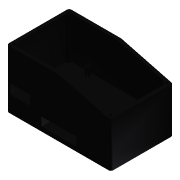
# Autodesk Inventor part: CustomBox_base
Saved by Autodesk Inventor 2013 (Build 170138000, 138)
## iProperties
Created: 2013-03-21
Part Number: CustomBox_base
Material: Generic
Document SubType Name: Modeling
Designer: Alexander
Density: 1 g/cm^3
Author: Alexander
Autodesk Inventor part; units mm, degrees
ref_plane "YZ Plane" through (0, 0, 0) normal (1, 0, 0) x (0, 1, 0)
ref_plane "XZ Plane" through (0, 0, 0) normal (0, 1, 0) x (-1, 0, 0)
sketch "Sketch1" plane through (0, 0, 0) normal (0, 1, 0) x (-1, 0, 0)
  line L0 (0, 0) -> (76.2, 0)
  line L1 (76.2, 0) -> (76.2, 45.72)
  line L2 (76.2, 45.72) -> (0, 45.72)
  line L3 (0, 45.72) -> (0, 0)
  dimension "d9" = 45.72
  dimension "d11" = 76.2
  constraints: 8 end point, 2 parallel, 1 horizontal, 1 perpendicular
  measures "d9" distance of L0.end L1.end
  measures "d11" distance of L1.end L2.end
extrude "Extrusion1" add sketch "Sketch1" along normal blind 2.54
sketch "Sketch5" plane through (0, 2.54, 0) normal (0, 1, 0) x (1, 0, 0)
  circle A0 centre (-57.15, -5.461) radius 1.5875
  circle A1 centre (-57.15, -40.259) radius 1.5875
  circle A2 centre (-6.35, -40.259) radius 1.5875
  circle A3 centre (-6.35, -5.461) radius 1.5875
  line L0 (0, 0) -> (-76.2, 0) projected
  line L1 (-76.2, 0) -> (-76.2, -45.72) projected
  line L2 (0, -45.72) -> (0, 0) projected
  line L3 (-76.2, -22.86) -> (0, -22.86)
  dimension "d8" = 3.175
  dimension "d12" = 3.175
  dimension "d13" = 3.175
  dimension "d14" = 3.175
  dimension "d15" = 34.798
  dimension "d16" = 50.8
  dimension "d32" = 5.461
  dimension "d34" = 6.35
  constraints: 4 centre point, 2 end point, 2 horizontal alignment, 2 midpoint, 2 vertical alignment
  measures "d8" diameter of A0
  measures "d12" diameter of A1
  measures "d13" diameter of A2
  measures "d14" diameter of A3
  measures "d15" distance of A1.centre A0.centre
  measures "d16" distance of A3.centre A0.centre
  measures "d32" distance from line of L0 A0.centre
  measures "d34" distance from line of L2 A2.centre
extrude "Extrusion4" add sketch "Sketch5" along normal blind 6.096 contours A0 | A1 | A2 | A3
sketch "Sketch6" plane through (0, 2.54, 0) normal (0, 1, 0) x (1, 0, 0)
  line L0 (-56.769, -39.624) -> (-6.985, -39.624)
  line L1 (-6.985, -39.624) -> (-6.985, -6.096)
  line L2 (-6.985, -6.096) -> (-56.769, -6.096)
  line L3 (-56.769, -6.096) -> (-56.769, -39.624)
  circle A0 centre (-57.15, -5.461) radius 1.5875 projected
  circle A1 centre (-57.15, -40.259) radius 1.5875 projected
  dimension "d21" = 49.784
  dimension "d22" = 33.528
  dimension "d25" = 0.381
  dimension "d27" = 0.635
  constraints: 8 end point, 2 parallel, 1 horizontal, 1 perpendicular
  measures "d21" distance of L2.end L1.end
  measures "d22" distance of L0.end L1.end
  measures "d25" distance from line of A0.centre L3
  measures "d27" distance from line of A1.centre L0
extrude "Extrusion6" cut sketch "Sketch6" along normal blind 6.35 contours L3 A1 L0 | A1 L3 A0 L2 L1 L0 | L3 L2 A0 picked at (-56.1138, -39.5193) picked at (-56.1138, -6.2007)
sketch "Sketch7" plane through (0, 2.54, 0) normal (0, 1, 0) x (1, 0, 0)
  line L0 (0, 0) -> (-76.2, 0) projected
  line L1 (-76.2, 0) -> (-76.2, -45.72) projected
  line L2 (-76.2, -45.72) -> (0, -45.72) projected
  line L3 (0, -45.72) -> (0, 0) projected
  line L4 (-72.205, -2.54) -> (-4.1275, -2.54)
  line L5 (-2.54, -4.1275) -> (-2.54, -41.5925)
  line L6 (-4.1275, -43.18) -> (-72.205, -43.18)
  line L7 (-73.66, -40.9575) -> (-73.66, -4.7625)
  arc A0 (-72.205, -43.18) -> (-73.66, -40.9575) centre (-73.66, -42.545) ccw
  arc A1 (-2.54, -41.5925) -> (-4.1275, -43.18) centre (-2.54, -43.18) ccw
  arc A2 (-4.1275, -2.54) -> (-2.54, -4.1275) centre (-2.54, -2.54) ccw
  arc A3 (-73.66, -4.7625) -> (-72.205, -2.54) centre (-73.66, -3.175) ccw
  dimension "d28" = 2.54
  dimension "d29" = 2.54
  dimension "d30" = 2.54
  dimension "d31" = 2.54
  dimension "d44" = 3.175
  dimension "d45" = 3.175
  dimension "d46" = 3.175
  dimension "d47" = 3.175
  constraints: 8 end point, 8 point on circle, 4 centre point, 2 parallel, 1 horizontal, 1 perpendicular
  measures "d28" distance between parallel lines of L0 L4
  measures "d29" distance between parallel lines of L7 L1
  measures "d30" distance between parallel lines of L2 L6
  measures "d31" distance between parallel lines of L3 L5
  measures "d44" diameter of A0
  measures "d45" diameter of A1
  measures "d46" diameter of A2
  measures "d47" diameter of A3
sketch "Sketch8" plane through (0, 8.636, 0) normal (0, 1, 0) x (1, 0, 0)
  arc A0 (-55.695, -6.096) -> (-56.769, -7.0021) centre (-57.15, -5.461) ccw projected
  arc A1 (-56.769, -38.7179) -> (-55.695, -39.624) centre (-57.15, -40.259) ccw projected
  arc A2 (-7.805, -39.624) -> (-6.985, -38.804) centre (-6.35, -40.259) ccw projected
  arc A3 (-6.985, -6.916) -> (-7.805, -6.096) centre (-6.35, -5.461) ccw projected
  point P0 (0, 0)
  constraints: 4 coincident
hole "Hole1" at (-57.15, 8.636, 5.461) at (-57.15, 8.636, 40.259) at (-6.35, 8.636, 40.259) at (-6.35, 8.636, 5.461) direction (0, -1, 0) diameter 1.6 depth 6.35 tip angle 118
fillet "Fillet1" radius 1.5875 3 edges at (0, 1.27, 45.72) (0, 1.27, 0) (-76.2, 1.27, 0)
fillet "Fillet2" radius 1.5875 1 edges at (-76.2, 1.27, 45.72)
extrude "Extrusion9" add sketch "Sketch7" along normal blind 30.48
sketch "Sketch13" plane through (-74.6125, 0, 45.72) normal (0, 0, 1) x (1, 0, 0)
  line L0 (0.9525, 9.74) -> (15.4525, 9.74)
  line L1 (15.4525, 9.74) -> (15.4525, 2.54)
  line L2 (15.4525, 2.54) -> (0.9525, 2.54)
  line L3 (0.9525, 2.54) -> (0.9525, 9.74)
  line L4 (-1.5875, 2.54) -> (-1.5875, 33.02) projected
  line L5 (0, 0) -> (73.025, 0) projected
  point P0 (74.6125, 0)
  dimension "d77" = 14.5
  dimension "d79" = 7.2
  dimension "d114" = 2.54
  dimension "d136" = 2.54
  constraints: 8 end point, 2 parallel, 1 horizontal, 1 perpendicular
  measures "d77" distance of L1.end L2.end
  measures "d79" distance between parallel lines of L2 L0
  measures "d114" distance between parallel lines of L3 L4
  measures "d136" distance between parallel lines of L5 L2
extrude "Extrusion12" cut sketch "Sketch13" against normal up to next
fillet "Fillet5" radius 1.5875 4 edges at (-76.2, 17.78, 45.72) (-76.2, 17.78, 0) (0, 17.78, 45.72) (0, 17.78, 0)
sketch "Sketch14" plane through (0, 0, 44.1325) normal (1, 0, 0) x (0, 0, -1)
  line L0 (0, 0) -> (42.545, 0) projected
  line L1 (-1.5346, 0) -> (-1.5346, -9.525)
  line L2 (-1.5346, -9.525) -> (44.1325, -9.525)
  line L3 (44.1325, -9.525) -> (44.1325, 0)
  line L4 (-1.5346, 0) -> (44.1325, 0)
  dimension "d85" = 9.525
  constraints: 8 end point, 3 perpendicular, 1 parallel
  measures "d85" distance of L1.start L1.end
extrude "Extrusion13" add sketch "Sketch14" against normal blind 76.2
fillet "Fillet6" radius 1.5875 4 edges at (0, -4.7625, 0) (0, -4.7625, 45.6671) (-76.2, -4.7625, 0) (-76.2, -4.7625, 45.6671)
sketch "Sketch16" plane through (-1.5875, 33.02, 0) normal (0, 0, -1) x (-1, 0, 0)
  line L0 (0, -42.545) -> (73.025, -42.545) projected
  line L1 (23.8125, -39.37) -> (49.2125, -39.37)
  line L2 (49.2125, -39.37) -> (49.2125, -33.02)
  line L3 (49.2125, -33.02) -> (23.8125, -33.02)
  line L4 (23.8125, -33.02) -> (23.8125, -39.37)
  line L5 (74.6125, -42.545) -> (74.6125, 0) projected
  point P0 (-1.5875, -33.02)
  dimension "d97" = 25.4
  dimension "d98" = 25.4
  dimension "d99" = 3.175
  dimension "d103" = 6.35
  constraints: 8 end point, 2 parallel, 1 horizontal, 1 perpendicular
  measures "d97" distance of L3.end L2.end
  measures "d98" distance between parallel lines of L5 L2
  measures "d99" distance between parallel lines of L0 L1
  measures "d103" distance of L3.end L1.start
extrude "Extrusion15" cut sketch "Sketch16" against normal through all
sketch "Sketch18" plane through (-1.5875, 33.02, 0) normal (0, 0, -1) x (-1, 0, 0)
  line L0 (-1.5875, 0) -> (-1.5875, -42.545) projected
  line L1 (74.6125, -42.545) -> (74.6125, 0) projected
  line L2 (12.7, 0) -> (74.6125, 0)
  line L3 (73.025, -16.3342) -> (74.6125, -16.3342)
  line L4 (-1.5875, -9.525) -> (-1.5875, -9.525)
  line L5 (-1.5875, 0) -> (36.5125, 0)
  line L6 (-1.5875, 0) -> (-1.5875, -9.525)
  line L7 (0, -42.545) -> (-1.5875, -42.545) projected
  line L8 (-1.5875, -9.525) -> (0, -9.525)
  line L9 (0, -9.525) -> (36.5125, 0)
  point P0 (-1.5875, -33.02)
  dimension "d110" = 38.1
  dimension "d135" = 9.525
  constraints: 14 end point, 2 collinear, 2 perpendicular, 2 point on line, 1 parallel
  measures "d110" distance from line of L1 L5.end
  measures "d135" distance between parallel lines of L8 L5
extrude "Extrusion23" cut sketch "Sketch18" against normal through all
sketch "Sketch23" plane through (0, 33.02, 0) normal (0, 1, 0) x (1, 0, 0)
  arc A0 (-72.205, -43.18) -> (-73.66, -40.9575) centre (-73.66, -42.545) ccw projected
  arc A1 (-73.66, -4.7625) -> (-72.205, -2.54) centre (-73.66, -3.175) ccw projected
  circle A2 centre (-73.66, -3.175) radius 0.7938
  circle A3 centre (-73.66, -42.545) radius 0.7937
  point P0 (0, 0)
  dimension "d137" = 1.5875
  dimension "d138" = 1.5875
  constraints: 2 centre point, 2 coincident
  measures "d137" diameter of A2
  measures "d138" diameter of A3
extrude "Extrusion24" cut sketch "Sketch23" against normal blind 6.35
ref_plane "Work Plane1" through (-1.5875, 25.0825, 45.72) normal (0, 1, 0) x (1, 0, 0)
sketch "Sketch26" plane through (-1.5875, 25.0825, 45.72) normal (0, 1, 0) x (1, 0, 0)
  arc A0 (-2.54, 43.18) -> (-0.9525, 41.5925) centre (-0.9525, 43.18) ccw projected
  circle A1 centre (-0.9525, 43.18) radius 0.7937
  arc A2 (-0.9525, 4.1275) -> (-2.54, 2.54) centre (-0.9525, 2.54) ccw projected
  circle A3 centre (-0.9525, 2.54) radius 0.7937
  point P0 (1.5875, 45.72)
  dimension "d142" = 1.5875
  dimension "d143" = 1.5875
  constraints: 2 centre point, 2 coincident
  measures "d142" diameter of A1
  measures "d143" diameter of A3
extrude "Extrusion25" cut sketch "Sketch26" against normal blind 6.35
equation "\"d32\" = -0.5 * d15 + 0.5 * d9"
body "Solid1"
